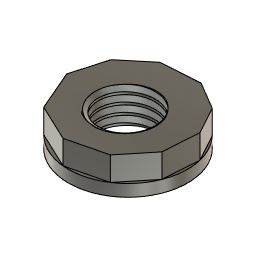
BoulonJoystick (Autodesk Fusion 360 design; units mm, degrees)
Autodesk Fusion 360 part; units mm, degrees
sketch "Esquisse1" plane through (0, 0, 0) normal (0, 0, 1) x (1, 0, 0)
  circle A0 centre (0.2063, 0.2759) radius 10
  line L0 (-18.3797, 0) -> (21.5999, 0)
  line L1 (9.5311, -3.3361) -> (9.9237, 2.6361)
  line L2 (-6.8856, -6.7743) -> (-0.7448, -9.6788)
  line L3 (0, 0) -> (-18.3797, 0)
  line L4 (-9.7899, 0) -> (-6.8856, -6.7743)
  circle A1 centre (0.2063, 0.2759) radius 5
  line L5 (9.9237, 2.6361) -> (7.42, 7.2014)
  line L6 (2.8137, 9.93) -> (-3.6731, 9.4928)
  line L7 (5.6366, -8.1212) -> (9.5311, -3.3361)
  line L8 (-0.7448, -9.6788) -> (5.6366, -8.1212)
  line L9 (-8.1431, 5.7794) -> (-9.7899, 0)
  line L10 (-3.6731, 9.4928) -> (-11.7791, 2.7588)
  line L11 (7.42, 7.2014) -> (2.8137, 9.93)
  dimension "d1" = 10
  dimension "d2" = 20
  constraint coincident L3.start origin
  constraint horizontal L3
  constraint parallel L0 L3
  constraint coincident L6.end A0
  constraint coincident L9.start A0
  constraint coincident L9.start L10
  constraint coincident L4.start A0
  constraint coincident L2.start A0
  constraint coincident L4.start L0
  constraint coincident L2.end A0
  constraint coincident L7.start A0
  constraint coincident L1.start A0
  constraint coincident L1.end A0
  constraint coincident L5.end A0
  constraint coincident L6.start A0
  measures "d1" diameter of A1
  measures "d2" diameter of A0
extrude "Extrusion1" add sketch "Esquisse1" against normal blind 6
extrude "Extrusion2" cut sketch "Esquisse1" against normal blind 4 contours A0 L0 L1 | A0 L5 | A0 L0 L1 | A0 L11 | A0 L7 | A0 L6 | A0 L8 | A0 L10 | A0 L2 | A0 L9 | A0 L4
extrude "Extrusion3" cut sketch "Esquisse1" against normal blind 21 contours L0 L3 A1 | L0 L3 A1
thread "Filetage1" "ISO Metric profile 11.0 M11x1.5 6H" major diameter 11.1933 minor diameter 9.5262 pitch 1.5 angle 60 modelled right hand crest width 0.4125 on face at (5.1814, -0.2219, -2) crest through (4.9694, 0.2759, -0.375)
